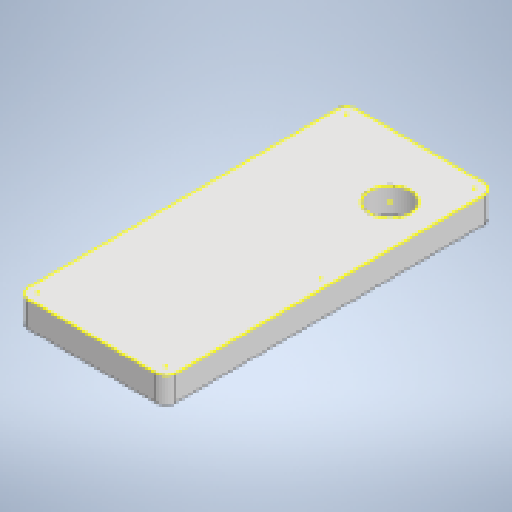
# Autodesk Inventor part: pcb_czujnik
Saved by Autodesk Inventor 2023 (Build 270158000, 158)
## iProperties
Created: 2025-01-15
Part Number: pcb_czujnik
Material: Ogólny
Document SubType Name: Modeling
Designer: kamil
Density: 1 g/cm^3
Appearance: Domyślna
Author: kamil
Autodesk Inventor part; units mm, degrees
ref_plane "YZ Plane" through (0, 0, 0) normal (1, 0, 0) x (0, 1, 0)
ref_plane "XZ Plane" through (0, 0, 0) normal (0, 1, 0) x (-1, 0, 0)
ref_plane "XY Plane" through (0, 0, 0) normal (0, 0, 1) x (1, 0, 0)
sketch "Szkic1" plane through (0, 0, 0) normal (0, 1, 0) x (-1, 0, 0)
  line L0 (8.4728, 9.9771) -> (-0.5272, 9.9771)
  line L1 (-0.5272, 9.9771) -> (-0.5272, -10.0229)
  line L2 (-0.5272, -10.0229) -> (8.4728, -10.0229)
  line L3 (8.4728, -10.0229) -> (8.4728, 9.9771)
  point P0 (0, 0)
  dimension "d0" = 9
  dimension "d1" = 20
  constraints: 8 end point, 2 parallel, 1 horizontal, 1 perpendicular
  measures "d0" distance of L2.end L1.end
  measures "d1" distance of L1.end L0.end
extrude "Wyciągnięcie proste1" add sketch "Szkic1" along normal blind 1.6
fillet "Zaokrąglenie1" radius 0.6 4 edges at (-8.4728, 0.8, -10.0229) (0.5272, 0.8, -10.0229) (0.5272, 0.8, 9.9771) (-8.4728, 0.8, 9.9771)
sketch "Szkic2" plane through (0, 0, 0) normal (0, -1, 0) x (1, 0, 0)
  circle A0 centre (-1.9728, -6.1673) radius 0.75 projected
  circle A1 centre (-1.9728, -6.1673) radius 1.25
  point P0 (0, 0)
  dimension "d5" = 2.5
  constraints: 1 centre point, 1 coincident
  measures "d5" diameter of A1
extrude "Wyciągnięcie proste2" cut sketch "Szkic2" against normal through all contours A0 | A1
